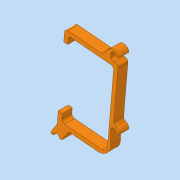
# Autodesk Inventor part: DriveBatteryHolder
Saved by Autodesk Inventor 2017 (Build 210142000, 142)
## iProperties
Created: 2018-01-31
Part Number: DriveBatteryHolder
Material: ABS Plastic
Document SubType Name: Modeling
Designer: Derek Wider
Density: 1.06 g/cm^3
Appearance: Orange
Author: Derek Wider
Autodesk Inventor part; units mm, degrees
ref_plane "YZ Plane" through (0, 0, 0) normal (1, 0, 0) x (0, 1, 0)
ref_plane "XZ Plane" through (0, 0, 0) normal (0, 1, 0) x (-1, 0, 0)
ref_plane "XY Plane" through (0, 0, 0) normal (0, 0, 1) x (1, 0, 0)
sketch "Sketch1" plane through (0, 0, 0) normal (0, 0, 1) x (1, 0, 0)
  arc A0 (1.905, 0) -> (-1.905, 0) centre (0, 0) ccw
  arc A1 (38.2001, 20.955) -> (34.3901, 20.9476) centre (36.2951, 20.955) ccw
  arc A2 (38.1877, 63.0819) -> (34.4025, 62.6481) centre (36.2951, 62.865) ccw
  line L0 (36.2951, 62.865) -> (36.2951, 20.955) construction
  line L1 (36.2951, 20.955) -> (0, 0) construction
  line L2 (32.146, 7.0452) -> (36.5038, 56.8549)
  line L3 (36.5038, 56.8549) -> (7.6142, 59.3825)
  line L4 (3.2564, 9.5727) -> (32.146, 7.0452)
  line L5 (0, 0) -> (62.4148, 0) construction
  line L6 (39.2555, 59.1639) -> (36.2181, 24.4467)
  line L7 (34.455, 4.2935) -> (7.7392, 6.6308)
  line L8 (7.1714, 54.3218) -> (4.6411, 54.5432)
  line L9 (3.6991, 14.6334) -> (1.1688, 14.8548)
  line L10 (38.2001, 20.955) -> (39.7876, 20.955)
  line L11 (-1.905, 0) -> (-3.4925, 0)
  line L12 (1.905, 0) -> (3.4925, 0)
  line L13 (0.5047, 7.2638) -> (1.1688, 14.8548)
  line L14 (4.6411, 54.5432) -> (5.3052, 62.1342)
  line L15 (7.6142, 59.3825) -> (7.1714, 54.3218)
  line L16 (3.6991, 14.6334) -> (3.2564, 9.5727)
  line L17 (0.5047, 7.2638) -> (-2.941, 1.8836)
  line L18 (3.4925, 0) -> (7.7392, 6.6308)
  line L19 (34.3901, 20.9476) -> (34.455, 4.2935)
  arc A3 (39.7876, 20.955) -> (36.2181, 24.4467) centre (36.2951, 20.955) ccw
  line L20 (33.6354, 65.1357) -> (29.2821, 60.0365)
  line L21 (38.1877, 63.0819) -> (39.7696, 63.2631)
  line L22 (34.4025, 62.6481) -> (34.7567, 59.5575)
  arc A4 (39.7696, 63.2631) -> (33.6354, 65.1357) centre (36.2951, 62.865) ccw
  arc A5 (-2.941, 1.8836) -> (-3.4925, 0) centre (0, 0) ccw
  line L23 (5.3052, 62.1342) -> (29.2821, 60.0365)
  line L24 (34.7567, 59.5575) -> (39.2555, 59.1639)
  dimension "d0" = 3.81
  dimension "d1" = 41.91
  dimension "d2" = 120
  dimension "d4" = 29
  dimension "d5" = 50
  dimension "d6" = 5.969
  dimension "d7" = 2.921
  dimension "d8" = 85
  dimension "d10" = 5.08
  dimension "d11" = 5.08
  dimension "d13" = 2.54
  constraints: 50 end point, 18 perpendicular, 12 point on circle, 6 centre point, 4 coincident, 4 tangent, 3 horizontal, 2 equal length, 2 equal radius, 2 point on line, 1 line through centre, 1 parallel, 1 vertical, 1 vertical alignment
  measures "d0" diameter of A0
  measures "d1" distance of L0.start L0.end
  measures "d2" angle of L0 L1
  measures "d4" distance of L4.start L2.start
  measures "d5" distance of L2.start L2.end
  measures "d6" distance from line of L3 L0.start
  measures "d7" distance from line of L2 L0.end
  measures "d8" angle of L5 L2
  measures "d10" distance between parallel lines of L8 L3
  measures "d11" distance between parallel lines of L4 L9
  measures "d13" distance between parallel lines of L14 L15
extrude "Extrusion1" add sketch "Sketch1" along normal blind 6.35
fillet "Fillet2" radius 3.175 1 edges at (32.146, 7.0452, 3.175)
fillet "Fillet1" radius 7.62 1 edges at (34.455, 4.2935, 3.175)
fillet "Fillet3" radius 1.905 10 edges at (3.2564, 9.5727, 3.175) (7.6142, 59.3825, 3.175) (36.5038, 56.8549, 3.175) (34.7567, 59.5575, 3.175) (29.2821, 60.0365, 3.175) (39.2555, 59.1639, 3.175) (36.2181, 24.4467, 3.175) (7.7392, 6.6308, 3.175) (0.5047, 7.2638, 3.175) (5.3052, 62.1342, 3.175)
equation "\"d13\" = d9"
equation "\"d9\" = 2.54"
body "Solid1"
